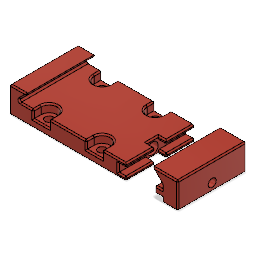
Quick Release Plate v9 (Autodesk Fusion 360 design; units mm, degrees)
Autodesk Fusion 360 part; units mm, degrees
note: some values were not read from the file. Set by a fixed rule: which face or edge a step refers to.
sketch "Sketch1" plane through (0, 0, 0) normal (0, 0, 1) x (1, 0, 0)
  line L0 (-22.015, 7) -> (-14.985, 7)
  line L1 (-14.985, 7) -> (-18.985, 3)
  line L2 (-18.985, 3) -> (22.015, 3)
  line L3 (22.015, 3) -> (22.015, -3)
  line L4 (22.015, -3) -> (-22.015, -3)
  line L5 (-22.015, -3) -> (-22.015, 7)
  line L6 (22.015, -1.5) -> (19.015, -1.5)
  line L7 (19.015, -1.5) -> (19.015, 1.5)
  line L8 (19.015, 1.5) -> (22.015, 1.5)
  line L9 (22.015, 1.5) -> (22.015, -1.5)
  line L10 (19.215, 1.3) -> (22.015, 1.3)
  line L11 (22.015, 1.3) -> (22.015, -1.3)
  line L12 (22.015, -1.3) -> (19.215, -1.3)
  line L13 (19.215, -1.3) -> (19.215, 1.3)
  line L14 (22.015, 1.3) -> (22.015, 3)
  line L15 (22.015, 3) -> (18.015, 7)
  line L16 (18.015, 7) -> (27.985, 7)
  line L17 (27.985, 7) -> (27.985, -3)
  line L18 (27.985, -3) -> (22.015, -3)
  dimension "d1" = 45
  dimension "d2" = 4
  dimension "d3" = 45
  dimension "d4" = 4
  dimension "d7" = 10
  dimension "d8" = 3
  dimension "d9" = 1.5
  dimension "d10" = 1.5
  dimension "d11" = 0.2
  dimension "d12" = 0.2
  dimension "d13" = 0.2
  dimension "d15" = 44.03
  dimension "d16" = 41
  dimension "d18" = 3
  dimension "d19" = 5.97
  dimension "d20" = 10
  dimension "d21" = 33
  dimension "d22" = 22.015
  measures "d1" angle of L1 L2
  measures "d2" distance of L0 L2
  measures "d3" angle of L2 L15
  measures "d4" distance of L2 L16
  measures "d9" distance of origin
  measures "d11" distance of L8 L10
  measures "d12" distance of L6 L12
  measures "d13" distance of L7 L13
  measures "d22" distance of origin L5
extrude "Extrude1" add sketch "Sketch1" along normal blind 26 contours L0 L1 L2 L3 L4 L5 L6 L7 L8 L14 makes body 1
extrude "Extrude2" add sketch "Sketch1" along normal blind 26 separate body contours L3 L9 L11 L14 L15 L16 L17 L18 | L3 L9 L10 L11 L12 L13 makes body 2
move_body "Move1" bodies 2 to x (1, 0, 0) y (0, 1, 0) z (0, 0, 1) at (0.5, 0, 0)
sketch "Sketch2" plane through (28.485, 0, 0) normal (1, 0, 0) x (0, 0, -1)
  line L0 (0, -3) -> (0, 7)
  line L1 (0, 7) -> (-26, 7)
  line L2 (-26, 7) -> (-26, -3)
  line L3 (-26, -3) -> (0, -3)
  circle A0 centre (-13, 0) radius 2.1
  circle A1 centre (-13, 0) radius 1.5
  dimension "d30" = 13
  dimension "d31" = 4.2
  dimension "d61" = 3
  measures "d30" distance of origin
  measures "d31" diameter of A0
  measures "d61" diameter of A1
extrude "Extrude3" cut sketch "Sketch2" against normal blind 8 from surface at -6.47 contours A0 | A1 bodies 1
sketch "Sketch3" plane through (0, 3, 0) normal (0, 1, 0) x (-1, 0, 0)
  line L0 (-22.015, 0) -> (18.985, 0)
  line L1 (18.985, 0) -> (18.985, 26)
  line L2 (18.985, 26) -> (-22.015, 26)
  line L3 (-22.015, 26) -> (-22.015, 0)
  line L4 (10, 3) -> (-10, 3) construction
  line L5 (-10, 3) -> (-10, 23) construction
  line L6 (-10, 23) -> (10, 23) construction
  line L7 (10, 23) -> (10, 3) construction
  circle A0 centre (10, 3) radius 1.5
  circle A1 centre (-10, 3) radius 1.5
  circle A2 centre (10, 23) radius 1.5
  circle A3 centre (-10, 23) radius 1.5
  circle A4 centre (10, 3) radius 3
  circle A5 centre (-10, 3) radius 3
  circle A6 centre (10, 23) radius 3
  circle A7 centre (-10, 23) radius 3
  line L8 (7, 3) -> (13, 3)
  line L9 (13, 3) -> (13, 0)
  line L10 (13, 0) -> (7, 0)
  line L11 (7, 0) -> (7, 3)
  line L12 (-7, 3) -> (-13, 3)
  line L13 (-13, 3) -> (-13, 0)
  line L14 (-13, 0) -> (-7, 0)
  line L15 (-7, 0) -> (-7, 3)
  line L16 (-13, 23) -> (-7, 23)
  line L17 (-7, 23) -> (-7, 26)
  line L18 (-7, 26) -> (-13, 26)
  line L19 (-13, 26) -> (-13, 23)
  line L20 (7, 23) -> (13, 23)
  line L21 (13, 23) -> (13, 26)
  line L22 (13, 26) -> (7, 26)
  line L23 (7, 26) -> (7, 23)
  dimension "d34" = 20
  dimension "d35" = 20
  dimension "d36" = 10
  dimension "d37" = 3
  dimension "d38" = 3
  dimension "d39" = 3
  dimension "d40" = 3
  dimension "d41" = 3
  dimension "d42" = 6
  dimension "d43" = 6
  dimension "d44" = 6
  dimension "d45" = 6
  dimension "d49" = 6
  dimension "d50" = 6
  dimension "d51" = 6
  dimension "d52" = 6
  measures "d36" distance of origin L5
  measures "d37" distance of origin L4
  measures "d38" diameter of A0
  measures "d39" diameter of A1
  measures "d40" diameter of A2
  measures "d41" diameter of A3
  measures "d42" diameter of A4
  measures "d43" diameter of A5
  measures "d44" diameter of A7
  measures "d45" diameter of A6
extrude "Extrude4" cut sketch "Sketch3" against normal through all contours A1 L12 | A1 L12 | A3 L16 | A3 L16 | A0 L8 | A0 L8 | A2 L20 | A2 L20 bodies 1
extrude "Extrude5" cut sketch "Sketch3" against normal blind 3 contours L0 A5 L13 L14 | L0 A5 L14 L15 | A1 A5 L12 | A1 A5 L12 | L2 A7 L18 L19 | L2 A7 L17 L18 | A3 A7 L16 | A3 A7 L16 | L0 A4 L10 L11 | L0 A4 L9 L10 | A0 A4 L8 | A0 A4 L8 | L2 A6 L22 L23 | L2 A6 L21 L22 | A2 A6 L20 | A2 A6 L20 bodies 1
sketch "Sketch4" plane through (22.015, 0, 0) normal (1, 0, 0) x (0, 0, -1)
  line L0 (-15.1, 3) -> (-10.9, 3)
  line L1 (-10.9, 3) -> (-10.9, -3)
  line L2 (-10.9, -3) -> (-15.1, -3)
  line L3 (-15.1, -3) -> (-15.1, 3)
  line L4 (0, -3) -> (-26, -3)
  circle A0 centre (-13, 0) radius 2.1
  arc A1 (-11.5303, 1.5) -> (-14.4697, 1.5) centre (-13, 0) ccw
  line L5 (-11.5303, 1.5) -> (0, 1.5)
  line L6 (0, 1.5) -> (0, 3)
  line L7 (0, 3) -> (-26, 3)
  line L8 (-26, 3) -> (-26, 1.5)
  line L9 (-26, 1.5) -> (-14.4697, 1.5)
  dimension "d57" = 4.2
  dimension "d78" = 6
  measures "d57" distance of L1 L3
  measures "d78" distance of L0 L2
extrude "Extrude6" cut sketch "Sketch4" against normal up to surface (3 mm away) contours L0 L1 L3 A0 A1 L5 L7 L9 | L3 A0 L9 | L1 A0 L5 | L1 L2 L3 L4 A0 bodies 1
extrude "Extrude7" cut sketch "Sketch2" against normal blind 9 contours A1 bodies 2
sketch "Sketch6" plane through (19.715, 0, 0) normal (-1, 0, 0) x (0, 0, 1)
  line L0 (10.9, 1.55) -> (15.1, 1.55)
  line L1 (15.1, 1.55) -> (15.1, -1.55)
  line L2 (15.1, -1.55) -> (10.9, -1.55)
  line L3 (10.9, -1.55) -> (10.9, 1.55)
  line L4 (13.7483, -1.3) -> (26, -1.3)
  line L5 (26, -1.3) -> (26, 1.3)
  line L6 (26, 1.3) -> (13.7483, 1.3)
  arc A0 (12.2517, 1.3) -> (12.2517, -1.3) centre (13, 0) ccw
  line L7 (12.2517, 1.3) -> (0, 1.3)
  line L8 (0, 1.3) -> (0, -1.3)
  line L9 (0, -1.3) -> (12.2517, -1.3)
  arc A1 (12.2517, -1.3) -> (13.7483, -1.3) centre (13, 0) ccw
  arc A2 (13.7483, 1.3) -> (12.2517, 1.3) centre (13, 0) ccw
  arc A3 (12.2517, 1.3) -> (12.2517, -1.3) centre (13, 0) ccw
  arc A4 (13.7483, -1.3) -> (13.7483, 1.3) centre (13, 0) ccw
  arc A5 (13.7483, -1.3) -> (13.7483, 1.3) centre (13, 0) ccw
  arc A6 (12.2517, 1.3) -> (12.2517, -1.3) centre (13, 0) ccw
  arc A7 (12.2517, 1.3) -> (12.2517, -1.3) centre (13, 0) ccw
  dimension "d71" = 2.1
  dimension "d72" = 4.2
  dimension "d76" = 3.1
  dimension "d77" = 1.55
  measures "d71" distance of L3
  measures "d77" distance of L0
extrude "Extrude10" cut sketch "Sketch6" against normal up to surface (2.8 mm away) contours L0 L1 L3 L6 L7 A2 | L3 A0 L7 L9 A3 A6 A7 | L1 L4 L6 A4 A5 | L1 L2 L3 L4 L9 A1 | A0 A1 A2 A3 A4 A5 A6 A7 bodies 2
move_body "Move2" bodies 2 to x (1, 0, 0) y (0, 1, 0) z (0, 0, 1) at (13, 0, 0)
fillet "Fillet4" radius 0.5 1 edges at (-18.985, 3, 13) on bodies 1
chamfer "Chamfer1" distance 0.5 angle 45 73 edges at (-22.015, 7, 13) (-22.015, 2, 26) (-18.5, 7, 26) (-14.985, 7, 13) (-18.5, 7, 0) (-13, 3, 24.5) (-10, 3, 20) (-7, 3, 24.5) (7, 3, 24.5) (10, 3, 20) (13, 3, 24.5) (13, 3, 1.5) (10, 3, 6) (7, 3, 1.5) (-7, 3, 1.5) (-10, 3, 6) (-13, 3, 1.5) (17.5075, 3, 26) (17.5075, 3, 0) (0, 3, 0) (0, 3, 26) (22.015, 3, 5.45) (22.015, 3, 20.55) (13, 1.5, 26) (10, 0, 26) (7, 1.5, 26) (-13, 1.5, 26) (-10, 0, 26) (-7, 1.5, 26) (19.015, 0, 26) (22.015, -2.25, 26) (20.515, -1.5, 26) (22.015, -1.5, 20.55) (22.015, -2.25, 15.1) (22.015, 1.5, 20.55) (20.515, 1.5, 26) (22.015, -2.25, 10.9) (22.015, -1.5, 5.45) (20.515, -1.5, 0) (22.015, -2.25, 0) (19.015, 0, 0) (22.015, 1.5, 5.45) (22.015, 2.25, 0) (20.515, 1.5, 0) (19.015, 3, 13) (-22.015, 2, 0) (-10, 0, 0) (-13, 1.5, 0) (-7, 1.5, 0) (7, 1.5, 0) (13, 1.5, 0) (10, 0, 0) (22.015, -3, 5.45) (0, -3, 0) (20.515, -1.5, 15.1) (20.515, -1.5, 10.9) (20.515, 1.5, 15.1) (20.515, 3, 15.1) (22.015, 2.25, 15.1) (20.515, 3, 10.9) (20.515, 1.5, 10.9) (20.515, -3, 15.1) (19.015, -3, 13) (22.015, -3, 20.55) (20.515, -3, 10.9) (-22.015, -3, 13) (0, -3, 26) (-15.3889, 3, 26) (-18.2398, 3.3087, 26) (-16.5582, 5.4268, 26) (-16.5582, 5.4268, 0) (-18.2398, 3.3087, 0) (-15.3889, 3, 0) on bodies 1
fillet "Fillet5" radius 0.5 1 edges at (35.515, 3, 13) on bodies 2
chamfer "Chamfer2" distance 0.5 angle 45 33 edges at (41.485, 7, 13) (36.5, 7, 0) (31.515, 7, 13) (36.5, 7, 26) (41.485, 2, 0) (34.115, 1.3, 0) (32.715, 1.3, 5.45) (32.715, 1.3, 20.55) (34.115, 1.3, 26) (41.485, 2, 26) (34.115, 1.3, 10.9) (34.115, 1.3, 15.1) (32.715, 0, 10.9) (34.115, -1.3, 10.9) (32.715, -1.3, 5.45) (32.715, 0, 15.1) (32.715, -1.3, 20.55) (32.715, 0, 26) (34.115, -1.3, 26) (35.515, -2.15, 26) (38.5, -3, 26) (34.115, -1.3, 0) (34.115, -1.3, 15.1) (35.515, -2.15, 0) (35.515, -3, 13) (38.5, -3, 0) (41.485, -3, 13) (33.4418, 5.0732, 26) (35.4769, 2.9842, 26) (35.515, 2.0464, 26) (35.515, 2.0464, 0) (35.4769, 2.9842, 0) (33.4418, 5.0732, 0) on bodies 2
equation "d22 = ( 44.03 / 2 ) * 1 mm"
